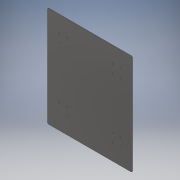
# Autodesk Inventor part: LiftBase
Saved by Autodesk Inventor 2018 (Build 220112000, 112)
## iProperties
Created: 2017-11-21
Part Number: LiftBase
Material: Steel, Galvanized
Document SubType Name: Modeling
Designer: P136265
Density: 7.85 g/cm^3
Appearance: Galvanized
Author: P136265
Autodesk Inventor part; units mm, degrees
ref_plane "YZ Plane" through (0, 0, 0) normal (1, 0, 0) x (0, 1, 0)
ref_plane "XZ Plane" through (0, 0, 0) normal (0, 1, 0) x (-1, 0, 0)
ref_plane "XY Plane" through (0, 0, 0) normal (0, 0, 1) x (1, 0, 0)
sketch "Sketch2" plane through (0, 0, 0) normal (0, 1, 0) x (-1, 0, 0)
  line L0 (-207.5, 252.5) -> (207.5, 252.5)
  line L1 (212.5, 247.5) -> (212.5, -247.5)
  line L2 (207.5, -252.5) -> (-207.5, -252.5)
  line L3 (-212.5, -247.5) -> (-212.5, 247.5)
  line L4 (-212.5, 252.5) -> (212.5, -252.5) construction
  line L5 (212.5, 252.5) -> (-212.5, -252.5) construction
  arc A0 (212.5, 247.5) -> (207.5, 252.5) centre (207.5, 247.5) ccw
  arc A1 (207.5, -252.5) -> (212.5, -247.5) centre (207.5, -247.5) ccw
  arc A2 (-207.5, 252.5) -> (-212.5, 247.5) centre (-207.5, 247.5) ccw
  arc A3 (-212.5, -247.5) -> (-207.5, -252.5) centre (-207.5, -247.5) ccw
  point P0 (0, 0)
  dimension "d10" = 425
  dimension "d11" = 505
  dimension "d12" = 5
  constraints: 12 end point, 8 point on circle, 8 point on line, 8 tangent, 4 centre point, 3 equal radius, 2 midpoint, 2 parallel, 1 horizontal, 1 perpendicular
  measures "d10" distance of L4.end L5.end
  measures "d11" distance of L5.start L4.end
  measures "d12" radius of A0
extrude "Extrusion3" add sketch "Sketch2" along normal mid plane 2
sketch "Sketch3" plane through (0, 1, 0) normal (0, 1, 0) x (1, 0, 0)
  line L0 (-212.5, 247.5) -> (-212.5, -247.5) construction
  arc A0 (-212.5, -247.5) -> (-207.5, -252.5) centre (-207.5, -247.5) ccw construction
  line L1 (-207.5, -252.5) -> (207.5, -252.5) construction
  arc A1 (207.5, -252.5) -> (212.5, -247.5) centre (207.5, -247.5) ccw construction
  line L2 (212.5, -247.5) -> (212.5, 247.5) construction
  arc A2 (212.5, 247.5) -> (207.5, 252.5) centre (207.5, 247.5) ccw construction
  line L3 (207.5, 252.5) -> (-207.5, 252.5) construction
  arc A3 (-207.5, 252.5) -> (-212.5, 247.5) centre (-207.5, 247.5) ccw construction
  circle A4 centre (-154.764, 129.6) radius 2.15 construction
  circle A5 centre (-154.764, 171.3) radius 2.15 construction
  circle A6 centre (-114.764, 129.6) radius 2.15 construction
  circle A7 centre (-114.764, 171.3) radius 2.15 construction
  circle A8 centre (114.764, 129.6) radius 2.15 construction
  circle A9 centre (114.764, 171.3) radius 2.15 construction
  circle A10 centre (154.764, 129.6) radius 2.15 construction
  circle A11 centre (154.764, 171.3) radius 2.15 construction
  line L4 (-212.5, 247.5) -> (-212.5, -247.5) construction
  line L5 (-212.5, 0) -> (212.5, 0) construction
  arc A12 (207.5, -252.5) -> (212.5, -247.5) centre (207.5, -247.5) ccw construction
  line L6 (207.5, -252.5) -> (-207.5, -252.5) construction
  arc A13 (-212.5, -247.5) -> (-207.5, -252.5) centre (-207.5, -247.5) ccw construction
  circle A14 centre (-154.764, -129.6) radius 2.15 construction
  circle A15 centre (-154.764, -171.3) radius 2.15 construction
  circle A16 centre (-114.764, -129.6) radius 2.15 construction
  circle A17 centre (-114.764, -171.3) radius 2.15 construction
  circle A18 centre (114.764, -129.6) radius 2.15 construction
  circle A19 centre (114.764, -171.3) radius 2.15 construction
  circle A20 centre (154.764, -129.6) radius 2.15 construction
  circle A21 centre (154.764, -171.3) radius 2.15 construction
  point P0 (0, 0)
  dimension "d15" = 4.3
  dimension "d16" = 4.3
  dimension "d17" = 41.7
  dimension "d18" = 81.2
  dimension "d19" = 57.736
  dimension "d20" = 4.3
  dimension "d21" = 97.736
  dimension "d22" = 4.3
  dimension "d23" = 4.3
  dimension "d24" = 327.264
  dimension "d25" = 4.3
  dimension "d26" = 4.3
  dimension "d27" = 367.264
  dimension "d28" = 4.3
  dimension "d29" = 41.7
  dimension "d30" = 41.7
  dimension "d31" = 81.2
  dimension "d32" = 81.2
  dimension "d33" = 57.736
  dimension "d34" = 97.736
  dimension "d35" = 327.264
  dimension "d36" = 81.2
  dimension "d37" = 122.9
  dimension "d38" = 367.264
  constraints: 18 centre point, 10 symmetric about line, 4 end point, 4 point on circle, 2 midpoint, 10 other
  measures "d15" diameter of A4
  measures "d16" diameter of A5
  measures "d17" distance of A4.centre A5.centre
  measures "d18" distance from line of L3 A5.centre
  measures "d19" distance from line of L0 A5.centre
  measures "d20" diameter of A6
  measures "d21" distance from line of L0 A6.centre
  measures "d22" diameter of A7
  measures "d23" diameter of A8
  measures "d24" distance from line of L0 A8.centre
  measures "d25" diameter of A9
  measures "d26" diameter of A10
  measures "d27" distance from line of L0 A10.centre
  measures "d28" diameter of A11
  measures "d29" distance of A9.centre A8.centre
  measures "d30" distance of A11.centre A10.centre
  measures "d31" distance from line of L3 A11.centre
  measures "d32" distance from line of L3 A9.centre
  measures "d33" distance from line of A11.centre L2
  measures "d34" distance from line of A9.centre L2
  measures "d35" distance from line of A7.centre L2
  measures "d36" distance from line of A7.centre L3
  measures "d37" distance from line of A6.centre L3
  measures "d38" distance from line of A4.centre L2
hole "Hole1" at (-154.764, 1, 171.3) at (-154.764, 1, 129.6) at (-114.764, 1, 129.6) at (-114.764, 1, 171.3) at (114.764, 1, 171.3) at (114.764, 1, 129.6) at (154.764, 1, 171.3) at (154.764, 1, 129.6) at (-154.764, 1, -171.3) at (-154.764, 1, -129.6) at (-114.764, 1, -129.6) at (-114.764, 1, -171.3) at (154.764, 1, -171.3) at (154.764, 1, -129.6) at (114.764, 1, -129.6) at (114.764, 1, -171.3) direction (0, -1, 0) diameter 4 end through all
body "Solid4"
